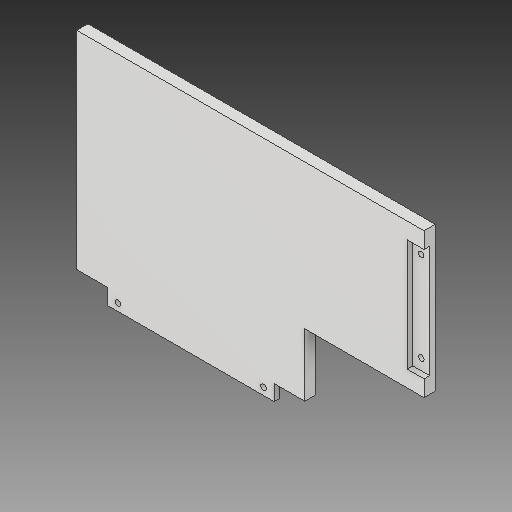
# Autodesk Inventor part: TC001b
Saved by Autodesk Inventor 2017 SP1 (Build 210196100, 196)
## iProperties
Created: 2018-01-07
Part Number: TC001b
Material: ABS Plastic
Document SubType Name: Modeling
Designer: Zach
Density: 1.06 g/cm^3
Appearance: CR White
Mass: 547.381 g
Surface Area: 1172.91 cm^2
Volume: 516.397 cm^3
Author: Zach
Autodesk Inventor part; units mm, degrees
ref_plane "YZ Plane" through (0, 0, 0) normal (1, 0, 0) x (0, 1, 0)
ref_plane "XZ Plane" through (0, 0, 0) normal (0, 1, 0) x (-1, 0, 0)
ref_plane "XY Plane" through (0, 0, 0) normal (0, 0, 1) x (1, 0, 0)
sketch "Sketch1" plane through (0, 0, 0) normal (0, 0, 1) x (1, 0, 0)
  line L0 (0, 0) -> (620, 0)
  line L1 (620, 0) -> (620, 620)
  line L2 (620, 620) -> (0, 620)
  line L3 (0, 620) -> (0, 0)
  line L4 (203.5, 491) -> (416.5, 491)
  line L5 (416.5, 491) -> (416.5, 378)
  line L6 (416.5, 378) -> (203.5, 378)
  line L7 (203.5, 378) -> (203.5, 491)
  point P0 (310, 491)
  point P1 (310, 620)
  dimension "d0" = 620
  dimension "d1" = 620
  dimension "d2" = 213
  dimension "d3" = 113
  dimension "d4" = 129
  constraints: 16 end point, 4 parallel, 2 horizontal, 2 midpoint, 2 perpendicular, 1 vertical alignment
  measures "d0" distance of L2.end L1.end
  measures "d1" distance of L1.end L0.end
  measures "d2" distance of L5.end L6.end
  measures "d3" distance of L4.end L5.end
  measures "d4" distance between parallel lines of L2 L4
extrude "Extrusion1" add sketch "Sketch1" along normal blind 10
sketch "Sketch2" plane through (0, 0, 10) normal (0, 0, 1) x (1, 0, 0)
  line L0 (0, 0) -> (310, 0)
  line L1 (310, 0) -> (310, 435)
  line L2 (310, 435) -> (0, 435)
  line L3 (0, 435) -> (0, 0)
  line L4 (620, 620) -> (0, 620) projected
  line L5 (0, 435) -> (620, 435)
  line L6 (620, 435) -> (620, 620)
  line L7 (620, 620) -> (0, 620)
  line L8 (0, 620) -> (0, 435)
  line L9 (310, 435) -> (620, 435)
  line L10 (620, 435) -> (620, 0)
  line L11 (620, 0) -> (310, 0)
  line L12 (310, 0) -> (310, 435)
  line L13 (620, 435) -> (310, 435)
  line L14 (310, 435) -> (310, 620)
  line L15 (310, 620) -> (620, 620)
  line L16 (620, 620) -> (620, 435)
  dimension "d7" = 435
  constraints: 32 end point, 8 parallel, 4 horizontal, 4 perpendicular, 1 midpoint, 1 vertical alignment
  measures "d7" distance of L1.end L0.end
extrude "Extrusion2" cut sketch "Sketch2" against normal through all contours L3 L2 L1 L0 | L1 L5 L10 L11 | L14 L4 L6 L5
sketch "Sketch6" plane through (0, 0, 10) normal (0, 0, 1) x (1, 0, 0)
  line L0 (310, 491) -> (310, 620) projected
  line L1 (310, 505.5) -> (295, 505.5)
  line L2 (295, 505.5) -> (295, 605.5)
  line L3 (295, 605.5) -> (310, 605.5)
  line L4 (310, 605.5) -> (310, 505.5)
  point P0 (0, 0)
  point P1 (310, 555.5)
  dimension "d30" = 15
  dimension "d31" = 100
  constraints: 8 end point, 2 midpoint, 2 parallel, 1 horizontal, 1 perpendicular, 1 point on line
  measures "d30" distance of L2.end L3.end
  measures "d31" distance of L1.end L2.end
extrude "Extrusion6" cut sketch "Sketch6" against normal blind 5
sketch "Sketch7" plane through (0, 0, 5) normal (0, 0, 1) x (1, 0, 0)
  line L0 (310, 605.5) -> (310, 505.5) construction
  line L1 (295, 605.5) -> (310, 605.5) construction
  line L2 (295, 505.5) -> (295, 605.5) construction
  line L3 (310, 505.5) -> (295, 505.5) construction
  circle A0 centre (302.5, 515.5) radius 2.5
  circle A1 centre (302.5, 595.5) radius 2.5
  point P0 (0, 0)
  point P1 (302.5, 605.5)
  point P2 (302.5, 505.5)
  dimension "d36" = 5
  dimension "d37" = 5
  dimension "d38" = 10
  dimension "d39" = 10
  constraints: 2 centre point, 2 midpoint, 2 vertical alignment
  measures "d36" diameter of A0
  measures "d37" diameter of A1
  measures "d38" distance from line of L1 A1.centre
  measures "d39" distance from line of L3 A0.centre
extrude "Extrusion7" cut sketch "Sketch7" against normal through all
sketch "Sketch8" plane through (0, 0, 10) normal (0, 0, 1) x (1, 0, 0)
  line L0 (203.5, 435) -> (0, 435) projected
  line L1 (27.25, 435) -> (176.25, 435)
  line L2 (176.25, 435) -> (176.25, 421)
  line L3 (176.25, 421) -> (27.25, 421)
  line L4 (27.25, 421) -> (27.25, 435)
  line L5 (26.75, 435) -> (176.75, 435) construction
  line L6 (176.75, 435) -> (176.75, 420) construction
  line L7 (176.75, 420) -> (26.75, 420) construction
  line L8 (26.75, 420) -> (26.75, 435) construction
  line L9 (0, 435) -> (203.5, 435) projected
  circle A0 centre (36.75, 427.5) radius 2.5
  circle A1 centre (166.75, 427.5) radius 2.5
  point P0 (0, 0)
  point P1 (101.75, 435)
  point P2 (101.75, 435)
  point P3 (176.75, 427.5)
  point P4 (26.75, 427.5)
  dimension "d44" = 149
  dimension "d45" = 14
  dimension "d46" = 150
  dimension "d47" = 15
  dimension "d48" = 5
  dimension "d49" = 5
  dimension "d50" = 10
  dimension "d51" = 10
  constraints: 16 end point, 6 midpoint, 4 parallel, 2 centre point, 2 horizontal, 2 horizontal alignment, 2 perpendicular, 1 point on line
  measures "d44" distance of L2.end L3.end
  measures "d45" distance of L1.end L2.end
  measures "d46" distance of L6.end L7.end
  measures "d47" distance of L5.end L6.end
  measures "d48" diameter of A0
  measures "d49" diameter of A1
  measures "d50" distance from line of L6 A1.centre
  measures "d51" distance from line of L8 A0.centre
extrude "Extrusion8" add sketch "Sketch8" against normal blind 5
body "Solid1"
